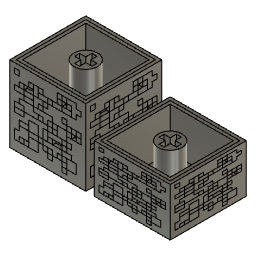
v2-Minecraft_ore_keycaps (Autodesk Fusion 360 design; units mm, degrees)
Autodesk Fusion 360 part; units mm, degrees
sketch "Sketch5" plane through (0, 0, 0) normal (0, 0, 1) x (1, 0, 0)
  line L0 (7.875, -1.125) -> (5.625, -1.125)
  line L1 (5.625, -1.125) -> (5.625, 0)
  line L2 (5.625, 0) -> (7.875, 0)
  line L3 (7.875, 0) -> (7.875, -1.125)
  line L4 (5.625, 1.125) -> (0, 1.125)
  line L5 (0, 1.125) -> (0, 2.25)
  line L6 (0, 2.25) -> (5.625, 2.25)
  line L7 (5.625, 2.25) -> (5.625, 1.125)
  line L8 (3.375, 2.25) -> (1.125, 2.25)
  line L9 (1.125, 2.25) -> (1.125, 3.375)
  line L10 (1.125, 3.375) -> (3.375, 3.375)
  line L11 (3.375, 3.375) -> (3.375, 2.25)
  line L12 (4.5, 5.625) -> (3.375, 5.625)
  line L13 (3.375, 5.625) -> (3.375, 6.75)
  line L14 (3.375, 6.75) -> (4.5, 6.75)
  line L15 (4.5, 6.75) -> (4.5, 5.625)
  line L16 (1.125, 4.5) -> (-1.125, 4.5)
  line L17 (-1.125, 4.5) -> (-1.125, 5.625)
  line L18 (-1.125, 5.625) -> (1.125, 5.625)
  line L19 (1.125, 5.625) -> (1.125, 4.5)
  line L20 (-2.25, 1.125) -> (-4.5, 1.125)
  line L21 (-4.5, 1.125) -> (-4.5, 3.375)
  line L22 (-4.5, 3.375) -> (-2.25, 3.375)
  line L23 (-2.25, 3.375) -> (-2.25, 1.125)
  line L24 (-4.5, 5.625) -> (-6.75, 5.625)
  line L25 (-6.75, 5.625) -> (-6.75, 6.75)
  line L26 (-6.75, 6.75) -> (-4.5, 6.75)
  line L27 (-4.5, 6.75) -> (-4.5, 5.625)
  line L28 (4.5, -3.375) -> (3.375, -3.375)
  line L29 (3.375, -3.375) -> (3.375, -2.25)
  line L30 (3.375, -2.25) -> (4.5, -2.25)
  line L31 (4.5, -2.25) -> (4.5, -3.375)
  line L32 (5.625, -6.75) -> (3.375, -6.75)
  line L33 (3.375, -6.75) -> (3.375, -5.625)
  line L34 (3.375, -5.625) -> (5.625, -5.625)
  line L35 (5.625, -5.625) -> (5.625, -6.75)
  line L36 (-1.1182, -6.75) -> (-3.375, -6.75)
  line L37 (-3.375, -6.75) -> (-3.375, -5.625)
  line L38 (-3.375, -5.625) -> (-1.1182, -5.625)
  line L39 (-1.1182, -5.625) -> (-1.1182, -6.75)
  line L40 (0, -5.625) -> (-6.75, -5.625)
  line L41 (-6.75, -5.625) -> (-6.75, -4.5)
  line L42 (-6.75, -4.5) -> (0, -4.5)
  line L43 (0, -4.5) -> (0, -5.625)
  line L44 (-3.375, -4.5) -> (-5.625, -4.5)
  line L45 (-5.625, -4.5) -> (-5.625, -3.375)
  line L46 (-5.625, -3.375) -> (-3.375, -3.375)
  line L47 (-3.375, -3.375) -> (-3.375, -4.5)
  line L48 (1.125, -2.25) -> (-3.375, -2.25)
  line L49 (-3.375, -2.25) -> (-3.375, -1.125)
  line L50 (-3.375, -1.125) -> (1.125, -1.125)
  line L51 (1.125, -1.125) -> (1.125, -2.25)
  line L52 (0, -1.125) -> (-2.25, -1.125)
  line L53 (-2.25, -1.125) -> (-2.25, 0)
  line L54 (-2.25, 0) -> (0, 0)
  line L55 (0, 0) -> (0, -1.125)
  line L56 (9, -9) -> (-9, -9)
  line L57 (-9, -9) -> (-9, 9)
  line L58 (-9, 9) -> (9, 9)
  line L59 (9, 9) -> (9, -9)
  constraint coincident L6 L8.start
  constraint midpoint L42 L44.start
  constraint coincident L50 L52.start
extrude "Extrude1" add sketch "Sketch5" along normal blind 0.75 makes body 1
copy_body "CopyPasteBodies1" bodies 1 makes body 2
move_body "Move1" bodies 2 to x (1, 0, 0) y (0, 0, 1) z (0, -1, 0) at (0, -4, 4)
move_body "Move2" bodies 2 to x (-1, 0, 0) y (0, 1, 0) z (0, 0, -1) at (0, 0, 8)
move_body "Move3" bodies 2 to x (1, 0, 0) y (0, 1, 0) z (0, 0, 1) at (0, -4.25, 5)
move_body "Move4" bodies 2 to x (-1, 0, 0) y (0, -1, 0) z (0, 0, 1) at (0, -18, 0)
move_body "Align1" bodies 2 to x (1, 0, 0) y (0, 1, 0) z (0, 0, 1) at (0, 0.75, 0)
pattern_circular "C-Pattern1" count 4 over 360 about axis through (0, 0, 1.75) along (0, 0, 1) of bodies 2 makes body 3 at (9, 7.5, 14.25) makes body 4 at (-7.5, 9, 14.25) makes body 5 at (-9, -7.5, 14.25)
combine "Combine1" operation add target body 1 tool bodies 2 3 4 5
sketch "Sketch7" plane through (0, 0, 0.75) normal (0, 0, 1) x (-1, 0, 0)
  line L0 (0, 0) -> (0, 1.125)
  line L1 (2.25, 0) -> (0, 0)
  line L2 (2.25, 1.125) -> (2.25, 0)
  line L3 (3.375, 1.125) -> (2.25, 1.125)
  line L4 (3.375, 2.25) -> (3.375, 1.125)
  line L5 (-1.125, 2.25) -> (3.375, 2.25)
  line L6 (-1.125, 1.125) -> (-1.125, 2.25)
  line L7 (0, 1.125) -> (-1.125, 1.125)
  line L8 (2.25, -3.375) -> (2.25, -1.125)
  line L9 (4.5, -3.375) -> (2.25, -3.375)
  line L10 (4.5, -1.125) -> (4.5, -3.375)
  line L11 (2.25, -1.125) -> (4.5, -1.125)
  line L12 (3.375, 3.375) -> (3.375, 4.5)
  line L13 (5.625, 3.375) -> (3.375, 3.375)
  line L14 (5.625, 4.5) -> (5.625, 3.375)
  line L15 (6.75, 4.5) -> (5.625, 4.5)
  line L16 (6.75, 5.625) -> (6.75, 4.5)
  line L17 (3.375, 5.625) -> (6.75, 5.625)
  line L18 (3.375, 6.75) -> (3.375, 5.625)
  line L19 (1.1182, 6.75) -> (3.375, 6.75)
  line L20 (1.1182, 5.625) -> (1.1182, 6.75)
  line L21 (0, 5.625) -> (1.1182, 5.625)
  line L22 (0, 4.5) -> (0, 5.625)
  line L23 (3.375, 4.5) -> (0, 4.5)
  line L24 (-4.5, 2.25) -> (-4.5, 3.375)
  line L25 (-3.375, 2.25) -> (-4.5, 2.25)
  line L26 (-3.375, 3.375) -> (-3.375, 2.25)
  line L27 (-4.5, 3.375) -> (-3.375, 3.375)
  line L28 (-5.625, 5.625) -> (-5.625, 6.75)
  line L29 (-3.375, 5.625) -> (-5.625, 5.625)
  line L30 (-3.375, 6.75) -> (-3.375, 5.625)
  line L31 (-5.625, 6.75) -> (-3.375, 6.75)
  line L32 (4.5, -6.75) -> (4.5, -5.625)
  line L33 (6.75, -6.75) -> (4.5, -6.75)
  line L34 (6.75, -5.625) -> (6.75, -6.75)
  line L35 (4.5, -5.625) -> (6.75, -5.625)
  line L36 (-1.125, -5.625) -> (-1.125, -4.5)
  line L37 (1.125, -5.625) -> (-1.125, -5.625)
  line L38 (1.125, -4.5) -> (1.125, -5.625)
  line L39 (-1.125, -4.5) -> (1.125, -4.5)
  line L40 (-4.5, -6.75) -> (-4.5, -5.625)
  line L41 (-3.375, -6.75) -> (-4.5, -6.75)
  line L42 (-3.375, -5.625) -> (-3.375, -6.75)
  line L43 (-4.5, -5.625) -> (-3.375, -5.625)
  line L44 (-3.375, -3.375) -> (-3.375, -2.25)
  line L45 (-1.125, -3.375) -> (-3.375, -3.375)
  line L46 (-1.125, -2.25) -> (-1.125, -3.375)
  line L47 (0, -2.25) -> (-1.125, -2.25)
  line L48 (0, -1.125) -> (0, -2.25)
  line L49 (-5.625, -1.125) -> (0, -1.125)
  line L50 (-5.625, -2.25) -> (-5.625, -1.125)
  line L51 (-3.375, -2.25) -> (-5.625, -2.25)
  line L52 (-7.875, 0) -> (-7.875, 1.125)
  line L53 (-5.625, 0) -> (-7.875, 0)
  line L54 (-5.625, 1.125) -> (-5.625, 0)
  line L55 (-7.875, 1.125) -> (-5.625, 1.125)
  circle A0 centre (0, 0) radius 2.8
  line L56 (8.25, -8.25) -> (8.25, 8.25)
  line L57 (8.25, 8.25) -> (-8.25, 8.25)
  line L58 (-8.25, 8.25) -> (-8.25, -8.25)
  line L59 (-8.25, -8.25) -> (8.25, -8.25)
  dimension "d12" = 5.6
  constraint coincident L1.start L0.start
  measures "d12" diameter of A0
extrude "Extrude2" add sketch "Sketch7" along normal blind 0.75 separate body contours L0 L1 L2 L3 L5 L6 L7 L8 L11 L46 L47 L48 L49 A0 | L0 L1 L2 L3 L5 L6 L7 A0 | L3 L4 L5 A0 | L44 L45 L46 L49 L50 L51 A0 | L46 L47 L48 L49 A0 | L8 L11 A0 | L8 L9 L10 L11 A0 | L12 L13 L14 L15 L16 L17 L18 L19 L20 L21 L22 L23 | L24 L25 L26 L27 | L28 L29 L30 L31 | L32 L33 L34 L35 | L36 L37 L38 L39 | L40 L41 L42 L43 | L52 L53 L54 L55 | L56 L57 L58 L59 makes body 6
extrude "Extrude3" add 1 faces at (2.75, 2.75, 1.5) along direction (0, 0, 1) blind 16.5 thin wall 0.75 inside separate body on bodies 6 makes body 7
extrude "Extrude4" add sketch "Sketch7" along normal blind 17.25 separate body contours L0 L1 L2 L3 L5 L6 L7 L8 L11 L46 L47 L48 L49 A0 | L0 L1 L2 L3 L5 L6 L7 A0 | L46 L47 L48 L49 A0 | L8 L11 A0 makes body 8
sketch "Sketch8" plane through (0, 0, 18) normal (0, 0, 1) x (-1, 0, 0)
  circle A0 centre (0, 0) radius 2.8
  line L0 (-0.585, 2.05) -> (0.585, 2.05)
  line L1 (0.585, -2.05) -> (-0.585, -2.05)
  line L2 (-0.585, 2.05) -> (0.585, -2.05) construction
  line L3 (0.585, 2.05) -> (-0.585, -2.05) construction
  line L4 (2.05, 0.585) -> (2.05, -0.585)
  line L5 (-2.05, -0.585) -> (-2.05, 0.585)
  line L6 (-2.05, 0.585) -> (2.05, -0.585) construction
  line L7 (2.05, 0.585) -> (-2.05, -0.585) construction
  line L8 (2.05, -0.585) -> (0.585, -0.585)
  line L9 (-0.585, -0.585) -> (-2.05, -0.585)
  line L10 (0.585, 2.05) -> (0.585, 0.585)
  line L11 (0.585, -0.585) -> (0.585, -2.05)
  line L12 (-2.05, 0.585) -> (-0.585, 0.585)
  line L13 (0.585, 0.585) -> (2.05, 0.585)
  line L14 (-0.585, -2.05) -> (-0.585, -0.585)
  line L15 (-0.585, 0.585) -> (-0.585, 2.05)
  dimension "d20" = 1.17
  dimension "d21" = 4.1
  dimension "d22" = 4.1
  dimension "d23" = 1.17
  constraint horizontal L0
  constraint perpendicular L0 L10
  constraint parallel L0 L1
  constraint parallel L10 L14
  constraint coincident L2 A0.centre
  constraint coincident L3 A0.centre
  constraint coincident A0.centre origin
  constraint horizontal L12
  constraint perpendicular L4 L12
  constraint parallel L8 L12
  constraint parallel L4 L5
  constraint coincident L6 A0.centre
  constraint coincident L7 A0.centre
  constraint collinear L8 L9
  constraint coincident L8.end L10
  constraint collinear L10 L11
  constraint coincident L10.end L12
  constraint collinear L12 L13
  constraint coincident L12.end L14
  constraint collinear L14 L15
  measures "d20" distance of L1.start L1.end
  measures "d21" distance of L0.end L1.start
  measures "d22" distance of L4.end L5.start
  measures "d23" distance of L4.start L4.end
extrude "Extrude5" cut sketch "Sketch8" against normal blind 8.5 contours L0 L1 L4 L5 L8 L9 L10 L11 L12 L13 L14 L15 bodies 8
combine "Combine3" operation add target body 7 tool bodies 6 8
sketch "Sketch9" plane through (0, 0, 0) normal (0, 0, 1) x (1, 0, 0)
  line L0 (9, 9) -> (-9, 9)
  line L1 (-9, 9) -> (-9, -9)
  line L2 (-9, -9) -> (9, -9)
  line L3 (9, -9) -> (9, 9)
  line L4 (9, 9) -> (-9, -9) construction
  line L5 (-9, 9) -> (9, -9) construction
  line L6 (-4.5, -4.5) -> (-6.75, -4.5)
  line L7 (-6.75, -4.5) -> (-6.75, -6.75)
  line L8 (-6.75, -6.75) -> (-4.5, -6.75)
  line L9 (-4.5, -6.75) -> (-4.5, -4.5)
  line L10 (-4.5, -4.5) -> (-6.75, -6.75) construction
  line L11 (-6.75, -4.5) -> (-4.5, -6.75) construction
  line L12 (4.5, -4.5) -> (2.25, -4.5)
  line L13 (2.25, -4.5) -> (2.25, -6.75)
  line L14 (2.25, -6.75) -> (4.5, -6.75)
  line L15 (4.5, -6.75) -> (4.5, -4.5)
  line L16 (4.5, -4.5) -> (2.25, -6.75) construction
  line L17 (2.25, -4.5) -> (4.5, -6.75) construction
  line L18 (-5.625, 2.25) -> (-7.875, 2.25)
  line L19 (-7.875, 2.25) -> (-7.875, 0)
  line L20 (-7.875, 0) -> (-5.625, 0)
  line L21 (-5.625, 0) -> (-5.625, 2.25)
  line L22 (-5.625, 2.25) -> (-7.875, 0) construction
  line L23 (-7.875, 2.25) -> (-5.625, 0) construction
  line L24 (-2.25, 7.875) -> (-4.5, 7.875)
  line L25 (-4.5, 7.875) -> (-4.5, 5.625)
  line L26 (-4.5, 5.625) -> (-2.25, 5.625)
  line L27 (-2.25, 5.625) -> (-2.25, 7.875)
  line L28 (-2.25, 7.875) -> (-4.5, 5.625) construction
  line L29 (-4.5, 7.875) -> (-2.25, 5.625) construction
  line L30 (7.875, 1.125) -> (5.625, 1.125)
  line L31 (5.625, 1.125) -> (5.625, -1.125)
  line L32 (5.625, -1.125) -> (7.875, -1.125)
  line L33 (7.875, -1.125) -> (7.875, 1.125)
  line L34 (7.875, 1.125) -> (5.625, -1.125) construction
  line L35 (5.625, 1.125) -> (7.875, -1.125) construction
  line L36 (-4.5, -2.25) -> (-3.375, -2.25)
  line L37 (-2.25, 0) -> (-2.25, 1.125)
  line L38 (-2.25, 1.125) -> (-4.5, 1.125)
  line L39 (-4.5, 1.125) -> (-4.5, -2.25)
  line L40 (-3.375, -3.375) -> (0, -3.375)
  line L41 (0, -3.375) -> (0, 0)
  line L42 (0, 0) -> (-2.25, 0)
  line L43 (-3.375, -2.25) -> (-3.375, -3.375)
  line L44 (5.625, 3.375) -> (5.625, 5.625)
  line L45 (0, 5.625) -> (0, 3.375)
  line L46 (1.125, 2.25) -> (3.375, 2.25)
  line L47 (3.375, 6.75) -> (2.25, 6.75)
  line L48 (0, 3.375) -> (1.125, 3.375)
  line L49 (3.375, 3.375) -> (5.625, 3.375)
  line L50 (1.125, 3.375) -> (1.125, 2.25)
  line L51 (5.625, 5.625) -> (3.375, 5.625)
  line L52 (1.125, 5.625) -> (0, 5.625)
  line L53 (3.375, 2.25) -> (3.375, 3.375)
  line L54 (3.375, 5.625) -> (3.375, 6.75)
  line L55 (1.125, 5.625) -> (2.25, 5.625)
  line L56 (2.25, 5.625) -> (2.25, 6.75)
  point P0 (-5.625, -5.625)
  point P1 (3.375, -5.625)
  point P2 (-6.75, 1.125)
  point P3 (-3.375, 6.75)
  point P4 (6.75, 0)
  constraint horizontal L0
  constraint perpendicular L0 L1
  constraint parallel L0 L2
  constraint parallel L1 L3
  constraint coincident L4 L41.end
  constraint coincident L5 L41.end
  constraint coincident L41.end L42.start
  constraint horizontal L6
  constraint perpendicular L6 L7
  constraint parallel L6 L8
  constraint parallel L7 L9
  constraint coincident L4 L6.start
  constraint coincident L10 P0
  constraint coincident L11 P0
  constraint coincident L4 P0
  constraint horizontal L12
  constraint perpendicular L12 L13
  constraint parallel L12 L14
  constraint parallel L13 L15
  constraint coincident L5 L12.start
  constraint coincident L16 P1
  constraint coincident L17 P1
  constraint horizontal L18
  constraint perpendicular L18 L19
  constraint parallel L18 L20
  constraint parallel L19 L21
  constraint coincident L22 P2
  constraint coincident L23 P2
  constraint horizontal L24
  constraint perpendicular L24 L25
  constraint parallel L24 L26
  constraint parallel L25 L27
  constraint coincident L28 P3
  constraint coincident L29 P3
  constraint horizontal L30
  constraint perpendicular L30 L31
  constraint parallel L30 L32
  constraint parallel L31 L33
  constraint coincident L34 P4
  constraint coincident L35 P4
  constraint horizontal L36
  constraint vertical L37
  constraint horizontal L38
  constraint vertical L39
  constraint horizontal L40
  constraint vertical L41
  constraint horizontal L42
  constraint vertical L43
  constraint midpoint L4 L41.end
  constraint coincident L4 L40.start
  constraint horizontal L48
  constraint vertical L44
  constraint horizontal L51
  constraint vertical L45
  constraint coincident L4 L44.end
  constraint horizontal L46
  constraint vertical L53
  constraint horizontal L47
  constraint coincident L4 L49.start
  constraint collinear L48 L49
  constraint coincident L52.start L51
  constraint coincident L51.end L53
  constraint collinear L51 L52
  constraint collinear L53 L54
  constraint horizontal L55
  constraint vertical L56
extrude "Extrude6" add sketch "Sketch9" along normal blind 0.75 separate body makes body 9
copy_body "CopyPasteBodies3" bodies 9 makes body 10
move_body "Move6" bodies 10 to x (1, 0, 0) y (0, 0, 1) z (0, -1, 0) at (0, -9, 9)
move_body "Align2" bodies 10 to x (1, 0, 0) y (0, 1, 0) z (0, 0, 1) at (0, 18, 0)
pattern_circular "C-Pattern2" count 4 over 360 about axis through (0, 0, 1.75) along (0, 0, 1) of bodies 10 makes body 11 at (-9, 7.125, 4.125) makes body 12 at (-7.125, -9, 4.125) makes body 13 at (9, -7.125, 4.125)
combine "Combine4" operation add target body 9 tool bodies 10 11 12 13
sketch "Sketch13" plane through (0, 0, 0) normal (0, 0, 1) x (1, 0, 0)
  line L0 (9, 9) -> (-9, 9)
  line L1 (-9, 9) -> (-9, -9)
  line L2 (-9, -9) -> (9, -9)
  line L3 (9, -9) -> (9, 9)
  line L4 (9, 9) -> (-9, -9) construction
  line L5 (-9, 9) -> (9, -9) construction
  line L6 (-4.5, -7.875) -> (-3.375, -7.875)
  line L7 (-3.375, -7.875) -> (-3.375, -6.75)
  line L8 (-3.375, -6.75) -> (-4.5, -6.75)
  line L9 (-4.5, -6.75) -> (-4.5, -7.875)
  line L10 (-6.75, 0) -> (-4.5, 0)
  line L11 (-4.5, 0) -> (-4.5, 2.25)
  line L12 (-4.5, 2.25) -> (-6.75, 2.25)
  line L13 (-6.75, 2.25) -> (-6.75, 0)
  line L14 (5.625, -1.125) -> (7.875, -1.125)
  line L15 (7.875, -1.125) -> (7.875, 0)
  line L16 (7.875, 0) -> (5.625, 0)
  line L17 (5.625, 0) -> (5.625, -1.125)
  line L18 (-1.125, 4.5) -> (0, 4.5)
  line L19 (0, 4.5) -> (0, 5.625)
  line L20 (0, 5.625) -> (-1.125, 5.625)
  line L21 (-1.125, 5.625) -> (-1.125, 4.5)
  line L22 (6.75, 6.75) -> (7.875, 6.75)
  line L23 (7.875, 6.75) -> (7.875, 7.875)
  line L24 (7.875, 7.875) -> (6.75, 7.875)
  line L25 (6.75, 7.875) -> (6.75, 6.75)
  line L26 (1.125, -5.625) -> (1.125, -1.125)
  line L27 (-1.125, -1.125) -> (1.125, -1.125)
  line L28 (-1.125, -1.125) -> (-1.125, 1.125)
  line L29 (-1.125, 1.125) -> (-2.25, 1.125)
  line L30 (-2.25, 1.125) -> (-2.25, -1.125)
  line L31 (-2.25, -1.125) -> (-3.375, -1.125)
  line L32 (-3.375, -1.125) -> (-3.375, -2.25)
  line L33 (-3.375, -2.25) -> (-4.5, -2.25)
  line L34 (-4.5, -2.25) -> (-4.5, -3.375)
  line L35 (-4.5, -3.375) -> (-3.375, -3.375)
  line L36 (-3.375, -4.5) -> (-2.25, -4.5)
  line L37 (-2.25, -4.5) -> (-2.25, -5.625)
  line L38 (-2.25, -5.625) -> (-1.125, -5.625)
  line L39 (-1.125, -5.625) -> (-1.125, -6.75)
  line L40 (-1.125, -6.75) -> (0, -6.75)
  line L41 (0, -6.75) -> (0, -5.625)
  line L42 (0, -5.625) -> (1.125, -5.625)
  line L43 (4.5, -5.625) -> (4.5, -3.375)
  line L44 (4.5, -3.375) -> (6.75, -3.375)
  line L45 (6.75, -3.375) -> (6.75, -4.5)
  line L46 (6.75, -4.5) -> (7.875, -4.5)
  line L47 (7.875, -4.5) -> (7.875, -6.75)
  line L48 (7.875, -6.75) -> (5.625, -6.75)
  line L49 (5.625, -6.75) -> (5.625, -5.625)
  line L50 (-3.375, -4.5) -> (-3.375, -3.375)
  line L51 (4.5, -5.625) -> (5.625, -5.625)
  line L52 (-6.75, 4.5) -> (-3.375, 4.5)
  line L53 (-3.375, 4.5) -> (-3.375, 5.625)
  line L54 (-3.375, 5.625) -> (-2.25, 5.625)
  line L55 (-2.25, 5.625) -> (-2.25, 6.75)
  line L56 (-2.25, 6.75) -> (-3.375, 6.75)
  line L57 (-3.375, 6.75) -> (-3.375, 7.875)
  line L58 (-3.375, 7.875) -> (-6.75, 7.875)
  line L59 (-6.75, 7.875) -> (-6.75, 6.75)
  line L60 (-7.875, 6.75) -> (-7.875, 5.625)
  line L61 (-7.875, 5.625) -> (-6.75, 5.625)
  line L62 (-6.75, 5.625) -> (-6.75, 4.5)
  line L63 (2.25, 2.25) -> (5.625, 2.25)
  line L64 (5.625, 2.25) -> (5.625, 3.375)
  line L65 (5.625, 3.375) -> (7.875, 3.375)
  line L66 (7.875, 3.375) -> (7.875, 4.5)
  line L67 (7.875, 4.5) -> (5.625, 4.5)
  line L68 (5.625, 4.5) -> (5.625, 5.625)
  line L69 (4.5, 5.625) -> (4.5, 6.75)
  line L70 (4.5, 6.75) -> (2.25, 6.75)
  line L71 (2.25, 6.75) -> (2.25, 4.5)
  line L72 (2.25, 4.5) -> (1.125, 4.5)
  line L73 (1.125, 4.5) -> (1.125, 3.375)
  line L74 (1.125, 3.375) -> (2.25, 3.375)
  line L75 (2.25, 3.375) -> (2.25, 2.25)
  line L76 (-7.875, 6.75) -> (-6.75, 6.75)
  line L77 (4.5, 5.625) -> (5.625, 5.625)
  constraint horizontal L0
  constraint perpendicular L0 L1
  constraint parallel L0 L2
  constraint parallel L1 L3
  constraint coincident L4 origin
  constraint coincident L5 origin
  constraint horizontal L6
  constraint vertical L7
  constraint horizontal L8
  constraint vertical L9
  constraint horizontal L10
  constraint vertical L11
  constraint horizontal L12
  constraint vertical L13
  constraint horizontal L14
  constraint vertical L15
  constraint horizontal L16
  constraint vertical L17
  constraint horizontal L18
  constraint vertical L19
  constraint horizontal L20
  constraint vertical L21
  constraint horizontal L22
  constraint vertical L23
  constraint horizontal L24
  constraint vertical L25
  constraint coincident L4 L23.end
  constraint coincident L4 L22.start
  constraint coincident L5 L26.end
  constraint perpendicular L6 L26
  constraint coincident L4 L27.start
  constraint perpendicular L26 L27
  constraint coincident L5 L28.end
  constraint perpendicular L27 L28
  constraint perpendicular L28 L29
  constraint perpendicular L29 L30
  constraint perpendicular L30 L31
  constraint perpendicular L31 L32
  constraint perpendicular L32 L33
  constraint perpendicular L33 L34
  constraint coincident L4 L35.end
  constraint perpendicular L34 L35
  constraint perpendicular L34 L36
  constraint perpendicular L36 L37
  constraint perpendicular L37 L38
  constraint perpendicular L38 L39
  constraint perpendicular L39 L40
  constraint perpendicular L40 L41
  constraint perpendicular L26 L42
  constraint perpendicular L27 L43
  constraint perpendicular L43 L44
  constraint perpendicular L44 L45
  constraint perpendicular L45 L46
  constraint perpendicular L46 L47
  constraint perpendicular L47 L48
  constraint coincident L5 L49.end
  constraint perpendicular L48 L49
  constraint perpendicular L35 L50
  constraint perpendicular L49 L51
  constraint parallel L14 L52
  constraint perpendicular L52 L53
  constraint perpendicular L53 L54
  constraint perpendicular L52 L55
  constraint perpendicular L55 L56
  constraint perpendicular L56 L57
  constraint perpendicular L57 L58
  constraint coincident L5 L59.end
  constraint perpendicular L56 L59
  constraint parallel L59 L60
  constraint perpendicular L60 L61
  constraint perpendicular L52 L62
  constraint coincident L4 L63.start
  constraint perpendicular L21 L63
  constraint perpendicular L63 L64
  constraint perpendicular L64 L65
  constraint perpendicular L65 L66
  constraint perpendicular L66 L67
  constraint coincident L4 L68.end
  constraint perpendicular L67 L68
  constraint perpendicular L67 L69
  constraint perpendicular L69 L70
  constraint perpendicular L70 L71
  constraint perpendicular L71 L72
  constraint perpendicular L72 L73
  constraint perpendicular L73 L74
  constraint perpendicular L63 L75
  constraint perpendicular L59 L76
  constraint perpendicular L68 L77
extrude "Extrude7" add sketch "Sketch13" along normal blind 0.75 separate body makes body 14
copy_body "CopyPasteBodies4" bodies 14 makes body 15
move_body "Move7" bodies 15 to x (1, 0, 0) y (0, 0, 1) z (0, -1, 0) at (0, -8.25, 9.75)
move_body "Align3" bodies 15 to x (1, 0, 0) y (0, 1, 0) z (0, 0, 1) at (0, 17.25, 0)
move_body "Align4" bodies 15 to x (1, 0, 0) y (0, 1, 0) z (0, 0, 1) at (0, 0, -0.75)
pattern_circular "C-Pattern3" count 4 over 360 about axis through (0, 0, 1.75) along (0, 0, 1) of bodies 15 makes body 16 at (-8.25, -6.75, 4.875) makes body 17 at (6.75, -9, 4.875) makes body 18 at (8.25, 6.75, 4.875)
combine "Combine5" operation add target body 14 tool bodies 15 16 17 18
sketch "Sketch14" plane through (0, 0, 0) normal (0, 0, 1) x (1, 0, 0)
  line L0 (9, 9) -> (-9, 9)
  line L1 (-9, 9) -> (-9, -9)
  line L2 (-9, -9) -> (9, -9)
  line L3 (9, -9) -> (9, 9)
  line L4 (9, 9) -> (-9, -9) construction
  line L5 (-9, 9) -> (9, -9) construction
  line L6 (-3.375, -5.625) -> (0, -5.625)
  line L7 (0, -5.625) -> (0, -4.5)
  line L8 (-3.375, -4.5) -> (-3.375, -5.625)
  line L9 (2.25, -4.5) -> (2.25, -3.375)
  line L10 (-5.625, -3.375) -> (-5.625, -4.5)
  line L11 (0, -3.375) -> (0, -2.25)
  line L12 (0, -2.25) -> (-4.5, -2.25)
  line L13 (-4.5, -2.25) -> (-4.5, -3.375)
  line L14 (4.5, -3.375) -> (6.75, -3.375)
  line L15 (6.75, -3.375) -> (6.75, -2.25)
  line L16 (6.75, -2.25) -> (4.5, -2.25)
  line L17 (4.5, -2.25) -> (4.5, -3.375)
  line L18 (-7.875, 0) -> (-5.625, 0)
  line L19 (-5.625, 1.125) -> (-5.625, 2.25)
  line L20 (-5.625, 2.25) -> (-7.875, 2.25)
  line L21 (-7.875, 2.25) -> (-7.875, 0)
  line L22 (-5.625, 0) -> (-4.5, 0)
  line L23 (-4.5, 0) -> (-4.5, 1.125)
  line L24 (-4.5, 1.125) -> (-5.625, 1.125)
  line L25 (1.125, 0) -> (7.875, 0)
  line L26 (7.875, 0) -> (7.875, 1.125)
  line L27 (1.125, 1.125) -> (1.125, 0)
  line L28 (6.75, 1.125) -> (6.75, 2.25)
  line L29 (6.75, 2.25) -> (3.375, 2.25)
  line L30 (3.375, 2.25) -> (3.375, 1.125)
  line L31 (-5.625, 4.5) -> (0, 4.5)
  line L32 (0, 4.5) -> (0, 5.625)
  line L33 (-5.625, 5.625) -> (-5.625, 4.5)
  line L34 (-2.25, 5.625) -> (-2.25, 6.75)
  line L35 (-2.25, 6.75) -> (-4.5, 6.75)
  line L36 (-4.5, 6.75) -> (-4.5, 5.625)
  line L37 (3.375, 4.5) -> (5.625, 4.5)
  line L38 (5.625, 4.5) -> (5.625, 5.625)
  line L39 (5.625, 5.625) -> (3.375, 5.625)
  line L40 (3.375, 5.625) -> (3.375, 4.5)
  line L41 (-5.625, -4.5) -> (-3.375, -4.5)
  line L42 (0, -4.5) -> (2.25, -4.5)
  line L43 (2.25, -3.375) -> (0, -3.375)
  line L44 (-4.5, -3.375) -> (-5.625, -3.375)
  line L45 (0, 5.625) -> (-2.25, 5.625)
  line L46 (-4.5, 5.625) -> (-5.625, 5.625)
  line L47 (7.875, 1.125) -> (6.75, 1.125)
  line L48 (3.375, 1.125) -> (1.125, 1.125)
  constraint horizontal L0
  constraint perpendicular L0 L1
  constraint parallel L0 L2
  constraint parallel L1 L3
  constraint coincident L4 origin
  constraint coincident L5 origin
  constraint horizontal L6
  constraint vertical L7
  constraint vertical L8
  constraint horizontal L41
  constraint vertical L9
  constraint horizontal L43
  constraint vertical L10
  constraint vertical L11
  constraint horizontal L12
  constraint vertical L13
  constraint coincident L13.end L43
  constraint horizontal L14
  constraint vertical L15
  constraint horizontal L16
  constraint vertical L17
  constraint horizontal L18
  constraint vertical L19
  constraint horizontal L20
  constraint vertical L21
  constraint horizontal L22
  constraint vertical L23
  constraint horizontal L24
  constraint horizontal L25
  constraint vertical L26
  constraint horizontal L47
  constraint vertical L27
  constraint vertical L28
  constraint horizontal L29
  constraint vertical L30
  constraint coincident L30.end L47
  constraint horizontal L31
  constraint vertical L32
  constraint horizontal L45
  constraint vertical L33
  constraint vertical L34
  constraint horizontal L35
  constraint vertical L36
  constraint coincident L36.end L45
  constraint horizontal L37
  constraint vertical L38
  constraint horizontal L39
  constraint vertical L40
  constraint coincident L4 L38.end
  constraint collinear L41 L42
  constraint collinear L43 L44
  constraint collinear L45 L46
  constraint collinear L47 L48
extrude "Extrude8" add sketch "Sketch14" along normal blind 0.75 separate body makes body 19
copy_body "CopyPasteBodies5" bodies 19 makes body 20
move_body "Move8" bodies 20 to x (1, 0, 0) y (0, 0, 1) z (0, -1, 0) at (0, -8.25, 9.75)
move_body "Move9" bodies 20 to x (1, 0, 0) y (0, 1, 0) z (0, 0, 1) at (0, 17.25, -0.75)
pattern_circular "C-Pattern4" count 4 over 360 about axis through (0, 0, 1.75) along (0, 0, 1) of bodies 20 makes body 21 at (-9, 0, 1.125) makes body 22 at (0, -9, 1.125) makes body 23 at (9, 0, 1.125)
combine "Combine6" operation add target body 19 tool bodies 20 21 22 23
copy_body "CopyPasteBodies6" bodies 7 makes body 24
move_face "OffsetFaces1" offset -6.6 3 faces at (-2.5, 8, 18) (-1.0742, 1.5132, 18) (0.195, -1.0733, 9.5) on bodies 24
copy_body "CopyPasteBodies7" bodies 1 makes body 25
scale "Scale2" factors (1, 1, 0.633333) about (9, 9, 18) bodies 25
move_face "OffsetFaces2" offset 0.275 1 faces at (7.25, -5, 7.075) on bodies 25
copy_body "CopyPasteBodies8" bodies 9 makes body 26
scale "Scale3" factors (1, 1, 0.633333) about (8.25, 0, 9) bodies 26
move_face "OffsetFaces3" offset 0.275 1 faces at (6.875, -4.625, 3.775) on bodies 26
copy_body "CopyPasteBodies9" bodies 14 makes body 27
scale "Scale4" factors (1, 1, 0.633333) about (-6.75, 9, 14.625) bodies 27
move_face "OffsetFaces4" offset 0.275 1 faces at (-6.5, -3.875, 5.8375) on bodies 27
copy_body "CopyPasteBodies10" bodies 19 makes body 28
scale "Scale5" factors (1, 1, 0.633333) about (-9, -9, 18) bodies 28
move_face "OffsetFaces5" offset 0.275 1 faces at (-1.125, 2.25, 7.075) on bodies 28
move_body "Move11" bodies 24 25 26 27 28 to x (1, 0, 0) y (0, 1, 0) z (0, 0, 1) at (20, 0, 0)
move_body "Align5" bodies 28 to x (1, 0, 0) y (0, 1, 0) z (0, 0, 1) at (0, 0, -6.6)
move_body "Align6" bodies 25 to x (1, 0, 0) y (0, 1, 0) z (0, 0, 1) at (0, 0, -6.6)
move_body "Align7" bodies 26 to x (1, 0, 0) y (0, 1, 0) z (0, 0, 1) at (0, 0, -3.3)
move_body "Align8" bodies 27 to x (1, 0, 0) y (0, 1, 0) z (0, 0, 1) at (0, 0, -5.3625)
equation "d54 = 11.4 / 18"
equation "d55 = 0.75 mm - 0.475 mm"
equation "d58 = 11.4 / 18"
equation "d59 = 0.75 mm - 0.475 mm"
equation "d62 = 11.4 / 18"
equation "d63 = 0.75 mm - 0.475 mm"
equation "d66 = 11.4 / 18"
equation "d67 = 0.75 mm - 0.475 mm"
named bodies: "diamond", "s1", "s1 (1)", "s1 (2)", "s1 (3)", "inner_stem", "stem", "emerald", "gold", "gold (1)", "gold (1) (1)", "gold (1) (2)", "gold (1) (3)", "redstone", "redstone (1)", "redstone (1) (1)", "redstone (1) (2)", "redstone (1) (3)", "stem_small", "diamond_small", "emerald_small", "gold_small", "redstone_small"
